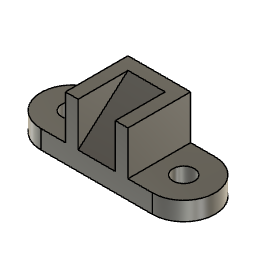
A2 (Autodesk Fusion 360 design; units mm, degrees)
Autodesk Fusion 360 part; units mm, degrees
sketch "Baza" plane through (0, 0, 0) normal (0, 0, 1) x (1, 0, 0)
  line L0 (57, 32) -> (-57, 32)
  line L1 (-57, -32) -> (57, -32)
  circle A0 centre (57, 0) radius 11
  circle A1 centre (-57, 0) radius 11
  arc A2 (57, -32) -> (57, 32) centre (57, 0) ccw
  arc A3 (-57, 32) -> (-57, -32) centre (-57, 0) ccw
  dimension "d1" = 114
  dimension "d2" = 64
  dimension "d3" = 22
  dimension "d4" = 22
  constraint horizontal L0
  constraint parallel L0 L1
  constraint concentric A0 A2
  constraint concentric A1 A3
  measures "d1" distance of L1.start L1.end
  measures "d2" distance of L0.end L1.start
  measures "d3" diameter of A0
  measures "d4" diameter of A1
extrude "Extrude1" add sketch "Baza" along normal blind 19
sketch "Pereti triunghi" plane through (0, 0, 19) normal (0, 0, 1) x (-1, 0, 0)
  circle A0 centre (57, 0) radius 11
  circle A1 centre (-57, 0) radius 11
  arc A2 (57, -32) -> (57, 32) centre (57, 0) ccw
  line L0 (57, 32) -> (-57, 32)
  arc A3 (-57, 32) -> (-57, -32) centre (-57, 0) ccw
  line L1 (-57, -32) -> (57, -32)
  line L2 (32, -32) -> (-32, -32)
  line L3 (32, -32) -> (32, 32)
  line L4 (-32, -32) -> (-32, 32)
  line L5 (19, -19) -> (-19, -19)
  line L6 (19, -19) -> (19, 32)
  line L7 (-19, -19) -> (-19, 32)
  dimension "d17" = 64
  dimension "d18" = 25
  dimension "d19" = 38
  dimension "d20" = 51
  dimension "d21" = 13
  constraint coincident L1 L2.start
  constraint parallel L1 L2
  constraint coincident L0 L3.end
  constraint perpendicular L0 L3
  constraint perpendicular L2 L4
  constraint perpendicular L4 L5
  constraint coincident L0 L6.end
  constraint perpendicular L0 L6
  constraint coincident L0 L7.end
  constraint perpendicular L0 L7
  measures "d17" distance of L2.start L2.end
  measures "d18" horizontal distance of A1.centre L2.end
  measures "d19" distance of L5.start L5.end
  measures "d20" distance of L0 L5
  measures "d21" distance of L4 L7
sketch "Triunghi" plane through (0, 0, 0) normal (1, 0, 0) x (0, 1, 0)
  line L0 (-32, 19) -> (19, 19)
  line L1 (19, 19) -> (19, 64)
  line L2 (-32, 19) -> (19, 64)
  dimension "d24" = 51
  dimension "d25" = 45
  constraint horizontal L0
  constraint perpendicular L0 L1
  measures "d24" distance of L0.start L0.end
  measures "d25" distance of L0.end L1.end
extrude "Extrude4" add sketch "Triunghi" along normal mid plane 38
extrude "Extrude5" add sketch "Pereti triunghi" along normal blind 45 contours L0 L1 L2 L3 L4 L5 L6 L7
equation "d18 = ( ( 114 - 64 ) / 2 ) * 1 mm"
equation "d21 = ( ( 64 - 38 ) / 2 ) * 1 mm"
equation "d25 = 64 mm - 19 mm"
equation "d28 = 64 mm - 19 mm"
named bodies: "A2"
